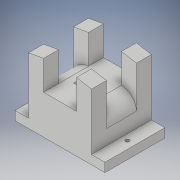
# Autodesk Inventor part: Foot_Ankl_Connector
Saved by Autodesk Inventor 2019 (Build 230136000, 136)
## iProperties
Created: 2018-06-02
Part Number: Foot_Ankl_Connector
Material: Generic
Document SubType Name: Modeling
Designer: Till
Density: 1 g/cm^3
Appearance: Default
Author: Till
Autodesk Inventor part; units mm, degrees
ref_plane "YZ Plane" through (0, 0, 0) normal (1, 0, 0) x (0, 1, 0)
ref_plane "XZ Plane" through (0, 0, 0) normal (0, 1, 0) x (-1, 0, 0)
ref_plane "XY Plane" through (0, 0, 0) normal (0, 0, 1) x (1, 0, 0)
sketch "Sketch1" plane through (0, 0, 0) normal (0, 0, 1) x (1, 0, 0)
  line L0 (-60, 0) -> (60, 0)
  line L1 (60, 0) -> (60, -52)
  line L2 (60, -52) -> (-60, -52)
  line L3 (-60, -52) -> (-60, 0)
  line L4 (0, -62.4) -> (0, 10.4) projected
  point P0 (0, 0)
  dimension "d0" = 120
  dimension "d1" = 52
  constraints: 8 end point, 2 parallel, 1 horizontal, 1 midpoint, 1 perpendicular, 1 other
  measures "d0" distance of L1.end L2.end
  measures "d1" distance of L2.end L0.start
extrude "Extrusion1" add sketch "Sketch1" along normal mid plane 80
sketch "Sketch2" plane through (-60, 0, 40) normal (0, 1, 0) x (1, 0, 0)
  line L0 (47.5, 49.5) -> (72.5, 49.5)
  line L1 (72.5, 49.5) -> (72.5, 30.5)
  line L2 (72.5, 30.5) -> (47.5, 30.5)
  line L3 (47.5, 30.5) -> (47.5, 49.5)
  line L4 (-24, 40) -> (144, 40) projected
  line L5 (60, 96) -> (60, -16) projected
  point P0 (60, 40)
  dimension "d4" = 19
  dimension "d5" = 25
  constraints: 8 end point, 2 parallel, 1 horizontal, 1 perpendicular, 2 other
  measures "d4" distance of L2.end L0.start
  measures "d5" distance of L0.start L0.end
extrude "Extrusion2" cut sketch "Sketch2" against normal blind 7
sketch "Sketch3" plane through (-60, 0, 40) normal (0, 1, 0) x (1, 0, 0)
  point P0 (60, 40)
  point P1 (60, 40)
  constraints: 1 coincident
hole "Hole1" at (0, 0, 0) direction (0, -1, 0) diameter 12 end through all
sketch "Sketch4" plane through (-60, 0, 40) normal (0, 1, 0) x (1, 0, 0)
  line L0 (-24, 40) -> (144, 40) projected
  line L1 (60, 96) -> (60, -16) projected
  point P0 (60, 40)
  point P1 (10, 40)
  point P2 (110, 40)
  dimension "d15" = 50
  constraints: 1 point on line, 1 symmetric about line
  measures "d15" distance of point (10, 40) point (60, 40)
hole "Hole2" at (-50, 0, 0) at (50, 0, 0) direction (0, -1, 0) diameter 5 end through all
sketch "Sketch5" plane through (0, 0, 0) normal (0, 0, 1) x (1, 0, 0)
  circle A0 centre (0, 43) radius 10.1 projected
  line L0 (0, 43) -> (42, 35.5943)
  line L1 (60, 0) -> (-60, 0) projected
  line L2 (42, 35.5943) -> (42, 0)
  line L3 (22, 0) -> (22, 39.1208)
  line L4 (22, 0) -> (42, 0)
  line L5 (0, -10.62) -> (0, 63.72) projected
  line L6 (0, 43) -> (-42, 35.5943)
  line L7 (-60, 0) -> (60, 0)
  line L8 (-42, 35.5943) -> (-42, 0)
  line L9 (-22, 0) -> (-22, 39.1208)
  point P0 (0, 0)
  dimension "d23" = 22
  dimension "d24" = 42
  dimension "d29" = 10
  constraints: 16 end point, 6 point on line, 6 symmetric about line, 1 collinear, 1 parallel, 1 perpendicular
  measures "d23" distance from line of L3 point (0, 0)
  measures "d24" distance from line of L2 point (0, 0)
  measures "d29" angle of L1 L0
extrude "Extrusion3" add sketch "Sketch5" along normal mid plane 80 contours L0 L2 L1 L3 | L9 L1 L8 L6
sketch "Sketch6" plane through (42, 0, 40) normal (1, 0, 0) x (0, 0, -1)
  line L0 (20, 0) -> (60, 0)
  line L1 (60, 0) -> (60, 44.1208)
  line L2 (60, 44.1208) -> (20, 44.1208)
  line L3 (20, 44.1208) -> (20, 0)
  line L4 (80, 35.5943) -> (80, 0) projected
  line L5 (0, 0) -> (0, 35.5943) projected
  line L6 (80, 39.1208) -> (0, 39.1208) projected
  point P0 (40, 0)
  dimension "d30" = 20
  dimension "d31" = 20
  dimension "d32" = 5
  constraints: 8 end point, 2 parallel, 1 horizontal, 1 perpendicular
  measures "d30" distance between parallel lines of L4 L1
  measures "d31" distance between parallel lines of L5 L3
  measures "d32" distance between parallel lines of L6 L2
extrude "Extrusion4" cut sketch "Sketch6" against normal through all
sketch "Sketch7" plane through (-60, 0, 40) normal (0, 1, 0) x (1, 0, 0)
  line L0 (0, 0) -> (0, 80) projected
  line L1 (18, 20) -> (18, 0) projected
  line L2 (0, 80) -> (18, 80)
  line L3 (18, 80) -> (18, 0)
  line L4 (18, 0) -> (0, 0)
  line L5 (0, 0) -> (0, 80)
  line L6 (120, 0) -> (102, 0) projected
  line L7 (102, 80) -> (102, 60) projected
  line L8 (120, 0) -> (102, 0)
  line L9 (102, 0) -> (102, 80)
  line L10 (102, 80) -> (120, 80)
  line L11 (120, 80) -> (120, 0)
  point P0 (60, 40)
  constraints: 16 end point, 4 parallel, 2 horizontal, 2 perpendicular
extrude "Extrusion5" cut sketch "Sketch7" against normal blind 40
fillet "Fillet1" radius 20 2 edges at (-42, 0, 0) (42, 0, 0)
equation "\"d31\" = d30"
body "Solid1"
